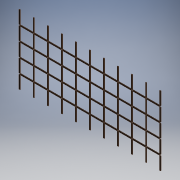
# Autodesk Inventor part: GridLedStructure
Saved by Autodesk Inventor 2017 (Build 210142000, 142)
## iProperties
Created: 2016-12-13
Part Number: GridLedStructure
Material: Bronze
Document SubType Name: Modeling
Designer: umr
Density: 8.47 g/cm^3
Appearance: Bronze - Polished
Author: umr
Autodesk Inventor part; units mm, degrees
ref_plane "YZ Plane" through (0, 0, 0) normal (1, 0, 0) x (0, 1, 0)
ref_plane "XZ Plane" through (0, 0, 0) normal (0, 1, 0) x (-1, 0, 0)
ref_plane "XY Plane" through (0, 0, 0) normal (0, 0, 1) x (1, 0, 0)
sketch "Sketch1" plane through (0, 0, 0) normal (0, 1, 0) x (-1, 0, 0)
  line L0 (0, 0) -> (20, 0)
  line L1 (20, 0) -> (20, -240)
  line L2 (20, -240) -> (0, -240)
  line L3 (0, -240) -> (0, 0)
  line L4 (0, 0) -> (0, -431.4913)
  line L5 (0, 0) -> (61.6406, 0)
  line L6 (20, -260) -> (20, -500)
  line L7 (0, -500) -> (0, -260)
  line L8 (20, -500) -> (0, -500)
  line L9 (0, -260) -> (20, -260)
  line L10 (20, -520) -> (20, -760)
  line L11 (0, -760) -> (0, -520)
  line L12 (20, -760) -> (0, -760)
  line L13 (0, -520) -> (20, -520)
  line L14 (20, -780) -> (20, -1020)
  line L15 (0, -1020) -> (0, -780)
  line L16 (20, -1020) -> (0, -1020)
  line L17 (0, -780) -> (20, -780)
  line L18 (20, -1040) -> (20, -1280)
  line L19 (0, -1280) -> (0, -1040)
  line L20 (20, -1280) -> (0, -1280)
  line L21 (0, -1040) -> (20, -1040)
  line L22 (-240, 0) -> (-240, -240)
  line L23 (-260, -240) -> (-260, 0)
  line L24 (-240, -240) -> (-260, -240)
  line L25 (-260, 0) -> (-240, 0)
  line L26 (-240, -260) -> (-240, -500)
  line L27 (-260, -500) -> (-260, -260)
  line L28 (-240, -500) -> (-260, -500)
  line L29 (-260, -260) -> (-240, -260)
  line L30 (-240, -520) -> (-240, -760)
  line L31 (-260, -760) -> (-260, -520)
  line L32 (-240, -760) -> (-260, -760)
  line L33 (-260, -520) -> (-240, -520)
  line L34 (-240, -780) -> (-240, -1020)
  line L35 (-260, -1020) -> (-260, -780)
  line L36 (-240, -1020) -> (-260, -1020)
  line L37 (-260, -780) -> (-240, -780)
  line L38 (-240, -1040) -> (-240, -1280)
  line L39 (-260, -1280) -> (-260, -1040)
  line L40 (-240, -1280) -> (-260, -1280)
  line L41 (-260, -1040) -> (-240, -1040)
  line L42 (-500, 0) -> (-500, -240)
  line L43 (-520, -240) -> (-520, 0)
  line L44 (-500, -240) -> (-520, -240)
  line L45 (-520, 0) -> (-500, 0)
  line L46 (-500, -260) -> (-500, -500)
  line L47 (-520, -500) -> (-520, -260)
  line L48 (-500, -500) -> (-520, -500)
  line L49 (-520, -260) -> (-500, -260)
  line L50 (-500, -520) -> (-500, -760)
  line L51 (-520, -760) -> (-520, -520)
  line L52 (-500, -760) -> (-520, -760)
  line L53 (-520, -520) -> (-500, -520)
  line L54 (-500, -780) -> (-500, -1020)
  line L55 (-520, -1020) -> (-520, -780)
  line L56 (-500, -1020) -> (-520, -1020)
  line L57 (-520, -780) -> (-500, -780)
  line L58 (-500, -1040) -> (-500, -1280)
  line L59 (-520, -1280) -> (-520, -1040)
  line L60 (-500, -1280) -> (-520, -1280)
  line L61 (-520, -1040) -> (-500, -1040)
  line L62 (-760, 0) -> (-760, -240)
  line L63 (-780, -240) -> (-780, 0)
  line L64 (-760, -240) -> (-780, -240)
  line L65 (-780, 0) -> (-760, 0)
  line L66 (-760, -260) -> (-760, -500)
  line L67 (-780, -500) -> (-780, -260)
  line L68 (-760, -500) -> (-780, -500)
  line L69 (-780, -260) -> (-760, -260)
  line L70 (-760, -520) -> (-760, -760)
  line L71 (-780, -760) -> (-780, -520)
  line L72 (-760, -760) -> (-780, -760)
  line L73 (-780, -520) -> (-760, -520)
  line L74 (-760, -780) -> (-760, -1020)
  line L75 (-780, -1020) -> (-780, -780)
  line L76 (-760, -1020) -> (-780, -1020)
  line L77 (-780, -780) -> (-760, -780)
  line L78 (-760, -1040) -> (-760, -1280)
  line L79 (-780, -1280) -> (-780, -1040)
  line L80 (-760, -1280) -> (-780, -1280)
  line L81 (-780, -1040) -> (-760, -1040)
  line L82 (-1020, 0) -> (-1020, -240)
  line L83 (-1040, -240) -> (-1040, 0)
  line L84 (-1020, -240) -> (-1040, -240)
  line L85 (-1040, 0) -> (-1020, 0)
  line L86 (-1020, -260) -> (-1020, -500)
  line L87 (-1040, -500) -> (-1040, -260)
  line L88 (-1020, -500) -> (-1040, -500)
  line L89 (-1040, -260) -> (-1020, -260)
  line L90 (-1020, -520) -> (-1020, -760)
  line L91 (-1040, -760) -> (-1040, -520)
  line L92 (-1020, -760) -> (-1040, -760)
  line L93 (-1040, -520) -> (-1020, -520)
  line L94 (-1020, -780) -> (-1020, -1020)
  line L95 (-1040, -1020) -> (-1040, -780)
  line L96 (-1020, -1020) -> (-1040, -1020)
  line L97 (-1040, -780) -> (-1020, -780)
  line L98 (-1020, -1040) -> (-1020, -1280)
  line L99 (-1040, -1280) -> (-1040, -1040)
  line L100 (-1020, -1280) -> (-1040, -1280)
  line L101 (-1040, -1040) -> (-1020, -1040)
  line L102 (-1280, 0) -> (-1280, -240)
  line L103 (-1300, -240) -> (-1300, 0)
  line L104 (-1280, -240) -> (-1300, -240)
  line L105 (-1300, 0) -> (-1280, 0)
  line L106 (-1280, -260) -> (-1280, -500)
  line L107 (-1300, -500) -> (-1300, -260)
  line L108 (-1280, -500) -> (-1300, -500)
  line L109 (-1300, -260) -> (-1280, -260)
  line L110 (-1280, -520) -> (-1280, -760)
  line L111 (-1300, -760) -> (-1300, -520)
  line L112 (-1280, -760) -> (-1300, -760)
  line L113 (-1300, -520) -> (-1280, -520)
  line L114 (-1280, -780) -> (-1280, -1020)
  line L115 (-1300, -1020) -> (-1300, -780)
  line L116 (-1280, -1020) -> (-1300, -1020)
  line L117 (-1300, -780) -> (-1280, -780)
  line L118 (-1280, -1040) -> (-1280, -1280)
  line L119 (-1300, -1280) -> (-1300, -1040)
  line L120 (-1280, -1280) -> (-1300, -1280)
  line L121 (-1300, -1040) -> (-1280, -1040)
  line L122 (-1540, 0) -> (-1540, -240)
  line L123 (-1560, -240) -> (-1560, 0)
  line L124 (-1540, -240) -> (-1560, -240)
  line L125 (-1560, 0) -> (-1540, 0)
  line L126 (-1540, -260) -> (-1540, -500)
  line L127 (-1560, -500) -> (-1560, -260)
  line L128 (-1540, -500) -> (-1560, -500)
  line L129 (-1560, -260) -> (-1540, -260)
  line L130 (-1540, -520) -> (-1540, -760)
  line L131 (-1560, -760) -> (-1560, -520)
  line L132 (-1540, -760) -> (-1560, -760)
  line L133 (-1560, -520) -> (-1540, -520)
  line L134 (-1540, -780) -> (-1540, -1020)
  line L135 (-1560, -1020) -> (-1560, -780)
  line L136 (-1540, -1020) -> (-1560, -1020)
  line L137 (-1560, -780) -> (-1540, -780)
  line L138 (-1540, -1040) -> (-1540, -1280)
  line L139 (-1560, -1280) -> (-1560, -1040)
  line L140 (-1540, -1280) -> (-1560, -1280)
  line L141 (-1560, -1040) -> (-1540, -1040)
  line L142 (-1800, 0) -> (-1800, -240)
  line L143 (-1820, -240) -> (-1820, 0)
  line L144 (-1800, -240) -> (-1820, -240)
  line L145 (-1820, 0) -> (-1800, 0)
  line L146 (-1800, -260) -> (-1800, -500)
  line L147 (-1820, -500) -> (-1820, -260)
  line L148 (-1800, -500) -> (-1820, -500)
  line L149 (-1820, -260) -> (-1800, -260)
  line L150 (-1800, -520) -> (-1800, -760)
  line L151 (-1820, -760) -> (-1820, -520)
  line L152 (-1800, -760) -> (-1820, -760)
  line L153 (-1820, -520) -> (-1800, -520)
  line L154 (-1800, -780) -> (-1800, -1020)
  line L155 (-1820, -1020) -> (-1820, -780)
  line L156 (-1800, -1020) -> (-1820, -1020)
  line L157 (-1820, -780) -> (-1800, -780)
  line L158 (-1800, -1040) -> (-1800, -1280)
  line L159 (-1820, -1280) -> (-1820, -1040)
  line L160 (-1800, -1280) -> (-1820, -1280)
  line L161 (-1820, -1040) -> (-1800, -1040)
  line L162 (-2060, 0) -> (-2060, -240)
  line L163 (-2080, -240) -> (-2080, 0)
  line L164 (-2060, -240) -> (-2080, -240)
  line L165 (-2080, 0) -> (-2060, 0)
  line L166 (-2060, -260) -> (-2060, -500)
  line L167 (-2080, -500) -> (-2080, -260)
  line L168 (-2060, -500) -> (-2080, -500)
  line L169 (-2080, -260) -> (-2060, -260)
  line L170 (-2060, -520) -> (-2060, -760)
  line L171 (-2080, -760) -> (-2080, -520)
  line L172 (-2060, -760) -> (-2080, -760)
  line L173 (-2080, -520) -> (-2060, -520)
  line L174 (-2060, -780) -> (-2060, -1020)
  line L175 (-2080, -1020) -> (-2080, -780)
  line L176 (-2060, -1020) -> (-2080, -1020)
  line L177 (-2080, -780) -> (-2060, -780)
  line L178 (-2060, -1040) -> (-2060, -1280)
  line L179 (-2080, -1280) -> (-2080, -1040)
  line L180 (-2060, -1280) -> (-2080, -1280)
  line L181 (-2080, -1040) -> (-2060, -1040)
  line L182 (-2320, 0) -> (-2320, -240)
  line L183 (-2340, -240) -> (-2340, 0)
  line L184 (-2320, -240) -> (-2340, -240)
  line L185 (-2340, 0) -> (-2320, 0)
  line L186 (-2320, -260) -> (-2320, -500)
  line L187 (-2340, -500) -> (-2340, -260)
  line L188 (-2320, -500) -> (-2340, -500)
  line L189 (-2340, -260) -> (-2320, -260)
  line L190 (-2320, -520) -> (-2320, -760)
  line L191 (-2340, -760) -> (-2340, -520)
  line L192 (-2320, -760) -> (-2340, -760)
  line L193 (-2340, -520) -> (-2320, -520)
  line L194 (-2320, -780) -> (-2320, -1020)
  line L195 (-2340, -1020) -> (-2340, -780)
  line L196 (-2320, -1020) -> (-2340, -1020)
  line L197 (-2340, -780) -> (-2320, -780)
  line L198 (-2320, -1040) -> (-2320, -1280)
  line L199 (-2340, -1280) -> (-2340, -1040)
  line L200 (-2320, -1280) -> (-2340, -1280)
  line L201 (-2340, -1040) -> (-2320, -1040)
  line L202 (0, -240) -> (-240, -240)
  line L203 (-240, -240) -> (-240, -260)
  line L204 (-240, -260) -> (0, -260)
  line L205 (0, -260) -> (0, -240)
  line L206 (-240, -520) -> (0, -520)
  line L207 (0, -520) -> (0, -500)
  line L208 (0, -500) -> (-240, -500)
  line L209 (-240, -500) -> (-240, -520)
  line L210 (-240, -780) -> (0, -780)
  line L211 (0, -780) -> (0, -760)
  line L212 (0, -760) -> (-240, -760)
  line L213 (-240, -760) -> (-240, -780)
  line L214 (-240, -1040) -> (0, -1040)
  line L215 (0, -1040) -> (0, -1020)
  line L216 (0, -1020) -> (-240, -1020)
  line L217 (-240, -1020) -> (-240, -1040)
  line L218 (-500, -260) -> (-260, -260)
  line L219 (-260, -260) -> (-260, -240)
  line L220 (-260, -240) -> (-500, -240)
  line L221 (-500, -240) -> (-500, -260)
  line L222 (-500, -520) -> (-260, -520)
  line L223 (-260, -520) -> (-260, -500)
  line L224 (-260, -500) -> (-500, -500)
  line L225 (-500, -500) -> (-500, -520)
  line L226 (-500, -780) -> (-260, -780)
  line L227 (-260, -780) -> (-260, -760)
  line L228 (-260, -760) -> (-500, -760)
  line L229 (-500, -760) -> (-500, -780)
  line L230 (-500, -1040) -> (-260, -1040)
  line L231 (-260, -1040) -> (-260, -1020)
  line L232 (-260, -1020) -> (-500, -1020)
  line L233 (-500, -1020) -> (-500, -1040)
  line L234 (-760, -260) -> (-520, -260)
  line L235 (-520, -260) -> (-520, -240)
  line L236 (-520, -240) -> (-760, -240)
  line L237 (-760, -240) -> (-760, -260)
  line L238 (-760, -520) -> (-520, -520)
  line L239 (-520, -520) -> (-520, -500)
  line L240 (-520, -500) -> (-760, -500)
  line L241 (-760, -500) -> (-760, -520)
  line L242 (-760, -780) -> (-520, -780)
  line L243 (-520, -780) -> (-520, -760)
  line L244 (-520, -760) -> (-760, -760)
  line L245 (-760, -760) -> (-760, -780)
  line L246 (-760, -1040) -> (-520, -1040)
  line L247 (-520, -1040) -> (-520, -1020)
  line L248 (-520, -1020) -> (-760, -1020)
  line L249 (-760, -1020) -> (-760, -1040)
  line L250 (-1020, -260) -> (-780, -260)
  line L251 (-780, -260) -> (-780, -240)
  line L252 (-780, -240) -> (-1020, -240)
  line L253 (-1020, -240) -> (-1020, -260)
  line L254 (-1020, -520) -> (-780, -520)
  line L255 (-780, -520) -> (-780, -500)
  line L256 (-780, -500) -> (-1020, -500)
  line L257 (-1020, -500) -> (-1020, -520)
  line L258 (-1020, -780) -> (-780, -780)
  line L259 (-780, -780) -> (-780, -760)
  line L260 (-780, -760) -> (-1020, -760)
  line L261 (-1020, -760) -> (-1020, -780)
  line L262 (-1020, -1040) -> (-780, -1040)
  line L263 (-780, -1040) -> (-780, -1020)
  line L264 (-780, -1020) -> (-1020, -1020)
  line L265 (-1020, -1020) -> (-1020, -1040)
  line L266 (-1280, -260) -> (-1040, -260)
  line L267 (-1040, -260) -> (-1040, -240)
  line L268 (-1040, -240) -> (-1280, -240)
  line L269 (-1280, -240) -> (-1280, -260)
  line L270 (-1280, -520) -> (-1040, -520)
  line L271 (-1040, -520) -> (-1040, -500)
  line L272 (-1040, -500) -> (-1280, -500)
  line L273 (-1280, -500) -> (-1280, -520)
  line L274 (-1280, -780) -> (-1040, -780)
  line L275 (-1040, -780) -> (-1040, -760)
  line L276 (-1040, -760) -> (-1280, -760)
  line L277 (-1280, -760) -> (-1280, -780)
  line L278 (-1280, -1040) -> (-1040, -1040)
  line L279 (-1040, -1040) -> (-1040, -1020)
  line L280 (-1040, -1020) -> (-1280, -1020)
  line L281 (-1280, -1020) -> (-1280, -1040)
  line L282 (-1540, -260) -> (-1300, -260)
  line L283 (-1300, -260) -> (-1300, -240)
  line L284 (-1300, -240) -> (-1540, -240)
  line L285 (-1540, -240) -> (-1540, -260)
  line L286 (-1540, -520) -> (-1300, -520)
  line L287 (-1300, -520) -> (-1300, -500)
  line L288 (-1300, -500) -> (-1540, -500)
  line L289 (-1540, -500) -> (-1540, -520)
  line L290 (-1540, -780) -> (-1300, -780)
  line L291 (-1300, -780) -> (-1300, -760)
  line L292 (-1300, -760) -> (-1540, -760)
  line L293 (-1540, -760) -> (-1540, -780)
  line L294 (-1540, -1040) -> (-1300, -1040)
  line L295 (-1300, -1040) -> (-1300, -1020)
  line L296 (-1300, -1020) -> (-1540, -1020)
  line L297 (-1540, -1020) -> (-1540, -1040)
  line L298 (-1800, -260) -> (-1560, -260)
  line L299 (-1560, -260) -> (-1560, -240)
  line L300 (-1560, -240) -> (-1800, -240)
  line L301 (-1800, -240) -> (-1800, -260)
  line L302 (-1800, -520) -> (-1560, -520)
  line L303 (-1560, -520) -> (-1560, -500)
  line L304 (-1560, -500) -> (-1800, -500)
  line L305 (-1800, -500) -> (-1800, -520)
  line L306 (-1800, -780) -> (-1560, -780)
  line L307 (-1560, -780) -> (-1560, -760)
  line L308 (-1560, -760) -> (-1800, -760)
  line L309 (-1800, -760) -> (-1800, -780)
  line L310 (-1800, -1040) -> (-1560, -1040)
  line L311 (-1560, -1040) -> (-1560, -1020)
  line L312 (-1560, -1020) -> (-1800, -1020)
  line L313 (-1800, -1020) -> (-1800, -1040)
  line L314 (-2060, -260) -> (-1820, -260)
  line L315 (-1820, -260) -> (-1820, -240)
  line L316 (-1820, -240) -> (-2060, -240)
  line L317 (-2060, -240) -> (-2060, -260)
  line L318 (-2060, -520) -> (-1820, -520)
  line L319 (-1820, -520) -> (-1820, -500)
  line L320 (-1820, -500) -> (-2060, -500)
  line L321 (-2060, -500) -> (-2060, -520)
  line L322 (-2060, -780) -> (-1820, -780)
  line L323 (-1820, -780) -> (-1820, -760)
  line L324 (-1820, -760) -> (-2060, -760)
  line L325 (-2060, -760) -> (-2060, -780)
  line L326 (-2060, -1040) -> (-1820, -1040)
  line L327 (-1820, -1040) -> (-1820, -1020)
  line L328 (-1820, -1020) -> (-2060, -1020)
  line L329 (-2060, -1020) -> (-2060, -1040)
  line L330 (-2320, -260) -> (-2080, -260)
  line L331 (-2080, -260) -> (-2080, -240)
  line L332 (-2080, -240) -> (-2320, -240)
  line L333 (-2320, -240) -> (-2320, -260)
  line L334 (-2320, -520) -> (-2080, -520)
  line L335 (-2080, -520) -> (-2080, -500)
  line L336 (-2080, -500) -> (-2320, -500)
  line L337 (-2320, -500) -> (-2320, -520)
  line L338 (-2320, -780) -> (-2080, -780)
  line L339 (-2080, -780) -> (-2080, -760)
  line L340 (-2080, -760) -> (-2320, -760)
  line L341 (-2320, -760) -> (-2320, -780)
  line L342 (-2320, -1040) -> (-2080, -1040)
  line L343 (-2080, -1040) -> (-2080, -1020)
  line L344 (-2080, -1020) -> (-2320, -1020)
  line L345 (-2320, -1020) -> (-2320, -1040)
  line L346 (-2580, -260) -> (-2340, -260)
  line L347 (-2340, -260) -> (-2340, -240)
  line L348 (-2340, -240) -> (-2580, -240)
  line L349 (-2580, -240) -> (-2580, -260)
  line L350 (-2580, -520) -> (-2340, -520)
  line L351 (-2340, -520) -> (-2340, -500)
  line L352 (-2340, -500) -> (-2580, -500)
  line L353 (-2580, -500) -> (-2580, -520)
  line L354 (-2580, -780) -> (-2340, -780)
  line L355 (-2340, -780) -> (-2340, -760)
  line L356 (-2340, -760) -> (-2580, -760)
  line L357 (-2580, -760) -> (-2580, -780)
  line L358 (-2580, -1040) -> (-2340, -1040)
  line L359 (-2340, -1040) -> (-2340, -1020)
  line L360 (-2340, -1020) -> (-2580, -1020)
  line L361 (-2580, -1020) -> (-2580, -1040)
  line L362 (-2580, 0) -> (-2580, -240)
  line L363 (-2600, -240) -> (-2600, 0)
  line L364 (-2580, -240) -> (-2600, -240)
  line L365 (-2600, 0) -> (-2580, 0)
  line L366 (-2580, -260) -> (-2580, -500)
  line L367 (-2600, -500) -> (-2600, -260)
  line L368 (-2580, -500) -> (-2600, -500)
  line L369 (-2600, -260) -> (-2580, -260)
  line L370 (-2580, -520) -> (-2580, -760)
  line L371 (-2600, -760) -> (-2600, -520)
  line L372 (-2580, -760) -> (-2600, -760)
  line L373 (-2600, -520) -> (-2580, -520)
  line L374 (-2580, -780) -> (-2580, -1020)
  line L375 (-2600, -1020) -> (-2600, -780)
  line L376 (-2580, -1020) -> (-2600, -1020)
  line L377 (-2600, -780) -> (-2580, -780)
  line L378 (-2580, -1040) -> (-2580, -1280)
  line L379 (-2600, -1280) -> (-2600, -1040)
  line L380 (-2580, -1280) -> (-2600, -1280)
  line L381 (-2600, -1040) -> (-2580, -1040)
  dimension "d0" = 20
  dimension "d1" = 240
  dimension "d4" = 260
  dimension "d7" = 260
  dimension "d12" = 260
  dimension "d15" = 260
  constraints: 764 end point, 5 horizontal, 4 parallel, 3 vertical, 2 perpendicular, 744 other
  measures "d0" distance of L1.end L2.end
  measures "d1" distance of L0.end L1.end
  measures "d4" distance of L0.end L6.start
  measures "d7" distance of L0.end L22.start
  measures "d12" distance of L26.start L206.start
  measures "d15" distance of L26.start L218.start
extrude "Extrusion1" add sketch "Sketch1" along normal blind 10 contours L21 L18 L20 L19 | L378 L380 L379 L381 | L364 L363 L365 L362 | L4 L204 L203 L202 | L0 L1 L2 L3 | L9 L6 L8 L7 L4 | L24 L23 L25 L22 | L26 L28 L27 L29 | L219 L218 L221 L220 | L207 L206 L209 L208 | L44 L43 L45 L42 | L13 L10 L12 L11 | L223 L222 L225 L224 | L30 L32 L31 L33 | L46 L48 L47 L49 | L235 L234 L237 L236 | L211 L210 L213 L212 | L64 L63 L65 L62 | L17 L14 L16 L15 | L227 L226 L229 L228 | L50 L52 L51 L53 | L239 L238 L241 L240 | L34 L36 L35 L37 | L66 L68 L67 L69 | L251 L250 L253 L252 | L215 L214 L217 L216 | L84 L83 L85 L82 | L231 L230 L233 L232 | L54 L56 L55 L57 | L243 L242 L245 L244 | L70 L72 L71 L73 | L255 L254 L257 L256 | L38 L40 L39 L41 | L86 L88 L87 L89 | L267 L266 L269 L268 | L104 L103 L105 L102 | L58 L60 L59 L61 | L247 L246 L249 L248 | L74 L76 L75 L77 | L259 L258 L261 L260 | L90 L92 L91 L93 | L271 L270 L273 L272 | L106 L108 L107 L109 | L283 L282 L285 L284 | L124 L123 L125 L122 | L78 L80 L79 L81 | L263 L262 L265 L264 | L94 L96 L95 L97 | L275 L274 L277 L276 | L110 L112 L111 L113 | L287 L286 L289 L288 | L126 L128 L127 L129 | L299 L298 L301 L300 | L144 L143 L145 L142 | L98 L100 L99 L101 | L279 L278 L281 L280 | L114 L116 L115 L117 | L291 L290 L293 L292 | L130 L132 L131 L133 | L303 L302 L305 L304 | L146 L148 L147 L149 | L315 L314 L317 L316 | L164 L163 L165 L162 | L118 L120 L119 L121 | L295 L294 L297 L296 | L134 L136 L135 L137 | L307 L306 L309 L308 | L150 L152 L151 L153 | L319 L318 L321 L320 | L166 L168 L167 L169 | L331 L330 L333 L332 | L184 L183 L185 L182 | L138 L140 L139 L141 | L311 L310 L313 L312 | L154 L156 L155 L157 | L323 L322 L325 L324 | L170 L172 L171 L173 | L335 L334 L337 L336 | L186 L188 L187 L189 | L347 L346 L349 L348 | L158 L160 L159 L161 | L327 L326 L329 L328 | L174 L176 L175 L177 | L339 L338 L341 L340 | L190 L192 L191 L193 | L351 L350 L353 L352 | L366 L368 L367 L369 | L178 L180 L179 L181 | L343 L342 L345 L344 | L194 L196 L195 L197 | L355 L354 L357 L356 | L370 L372 L371 L373 | L198 L200 L199 L201 | L359 L358 L361 L360 | L374 L376 L375 L377
equation "\"d4\" = d1 + d0"
equation "\"d7\" = d4"
equation "\"d12\" = d4"
equation "\"d15\" = d4"
body "Solid1"
